Shaft v5 (Autodesk Fusion 360 design; units mm, degrees)
Autodesk Fusion 360 part; units mm, degrees
sketch "Sketch1" plane through (0, 0, 0) normal (0, 0, 1) x (1, 0, 0) in component "Normalny"
  circle A0 centre (0, 0) radius 6
  circle A1 centre (0, -1) radius 6 construction
  line L0 (0, 0) -> (0, -7) construction
  line L1 (0, 0) -> (-6, 0) construction
  line L2 (0, 0) -> (6, 0) construction
  circle A2 centre (-3, 0) radius 1.55
  circle A3 centre (3, 0) radius 1.55
  circle A4 centre (0, 0) radius 7
  dimension "d1" = 12
  dimension "d2" = 12
  dimension "d3" = 1
  dimension "d13" = 3.1
  dimension "d14" = 3.1
  dimension "d20" = 1
  dimension "d78" = 6
  dimension "d79" = 3
  constraint coincident A0.centre L0.start
  constraint coincident A0 L1.end
  constraint horizontal L1
  constraint coincident A0 L2.end
  constraint parallel L1 L2
  constraint coincident L1 A2.centre
  constraint coincident L2 A3.centre
  constraint perpendicular L0 L2
  measures "d1" diameter of A0
  measures "d2" diameter of A1
  measures "d3" distance of A0.centre A1.centre
  measures "d13" diameter of A2
  measures "d14" diameter of A3
  measures "d78" distance of A2.centre A3.centre
  measures "d79" distance of A0.centre A2.centre
extrude "Extrude1" add sketch "Sketch1" along normal blind 7 contours A0 makes body 1 in component "Normalny"
extrude "Extrude2" add sketch "Sketch1" along normal blind 3 contours A4 bodies 1 in component "Normalny"
sketch "Sketch1 (2)" plane through (0, 0, 0) normal (0, 0, -1) x (1, 0, 0) in component "Shifted"
  circle A0 centre (0, 0) radius 7
  circle A1 centre (-3, 0) radius 1.55
  circle A2 centre (3, 0) radius 1.55
  circle A3 centre (0, -1) radius 6
  line L0 (0, 0) -> (0, -3) construction
  dimension "d23" = 12
  dimension "d24" = 1
  constraint coincident A0.centre L0.start
  constraint vertical L0
  measures "d23" diameter of A3
  measures "d24" distance of A3.centre A0.centre
extrude "Extrude1'" add sketch "Sketch1 (2)" along normal blind 7 separate body contours A3 makes body 2 in component "Shifted"
sketch "Sketch2" plane through (0, 0, -7) normal (0, 0, -1) x (1, 0, 0) in component "Shifted"
  circle A0 centre (3, 0) radius 1.55
  circle A1 centre (-3, 0) radius 1.55
  circle A2 centre (0, -1) radius 6
  circle A3 centre (0, -1) radius 7
  dimension "d27" = 1
extrude "Extrude2'" add sketch "Sketch2" against normal blind 3 contours A3 bodies 2 in component "Shifted"
sketch "Sketch1 (3)" plane through (0, 0, -7) normal (0, 0, -1) x (1, 0, 0) in component "Shifted_2"
  circle A0 centre (0, -1) radius 7
  circle A1 centre (3, 0) radius 1.55
  circle A2 centre (-3, 0) radius 1.55
  line L0 (0, 0) -> (0, 4) construction
  circle A3 centre (0, 1) radius 6
  dimension "d30" = 12
  dimension "d31" = 1
  constraint coincident L0.start origin
  constraint vertical L0
  constraint coincident L0 A3.centre
  measures "d30" diameter of A3
  measures "d31" distance of L0.start A3.centre
extrude "Extrude1''" add sketch "Sketch1 (3)" along normal blind 7 separate body contours A0 A3 | A0 A3 picked at (0.1647, 2.697) picked at (0, 6.3217) makes body 3 in component "Shifted_2"
sketch "Sketch2 (2)" plane through (0, 0, -14) normal (0, 0, -1) x (1, 0, 0) in component "Shifted_2"
  circle A0 centre (-3, 0) radius 1.55
  circle A1 centre (3, 0) radius 1.55
  circle A2 centre (0, 1) radius 6
  circle A3 centre (0, 1) radius 7
  dimension "d73" = 1
extrude "Extrude2''" add sketch "Sketch2 (2)" against normal blind 3 contours A3 bodies 3 in component "Shifted_2"
sketch "Sketch1 (4)" plane through (0, 0, -14) normal (0, 0, -1) x (1, 0, 0) in component "normalny2"
  circle A0 centre (0, 0) radius 6
  circle A1 centre (0, 1) radius 7
  circle A2 centre (-3, 0) radius 1.55
  circle A3 centre (3, 0) radius 1.55
  dimension "d37" = 12
  constraint coincident A0.centre origin
  measures "d37" diameter of A0
extrude "Extrude1'''" add sketch "Sketch1 (4)" along normal blind 4 separate body contours A0 makes body 4 in component "normalny2"
sketch "Sketch2 (3)" plane through (0, 0, 0) normal (0, 0, -1) x (1, 0, 0) in component "Normalny"
  circle A0 centre (0, 0) radius 7
  circle A1 centre (-3, 0) radius 1.55
  circle A2 centre (3, 0) radius 1.55
  circle A3 centre (0, -1) radius 6
  circle A4 centre (0, -1) radius 7
  dimension "d40" = 1
sketch "Sketch3" plane through (0, 0, -7) normal (0, 0, -1) x (1, 0, 0) in component "Shifted"
  circle A0 centre (0, -1) radius 7
  circle A1 centre (3, 0) radius 1.55
  circle A2 centre (-3, 0) radius 1.55
  circle A3 centre (0, 1) radius 7
  circle A4 centre (0, 1) radius 6
  constraint concentric A3 A4
extrude "Extrude3" add sketch "Sketch3" along normal blind 3 contours A0 A3 A4 | A0 A3 A4 | A0 A4 | A0 A4 bodies 2 in component "Shifted"
extrude "Extrude3'" add sketch "Sketch2 (3)" along normal blind 3 contours A3 | A0 A4 | A0 A4 picked at (1.4828, 5.4862) picked at (0.6054, -7.293) bodies 1 in component "Normalny"
sketch "Sketch4" plane through (0, 0, -14) normal (0, 0, -1) x (1, 0, 0) in component "Shifted_2"
  circle A0 centre (0, 0) radius 6
  circle A1 centre (0, 0) radius 7
  circle A2 centre (0, 1) radius 7
  circle A3 centre (-3, 0) radius 1.55
  circle A4 centre (3, 0) radius 1.55
  dimension "d62" = 1
extrude "Extrude4" add sketch "Sketch4" along normal blind 3 contours A0 | A1 A2 | A1 A2 picked at (1.4828, 6.4862) picked at (0.6054, -6.293) bodies 3 in component "Shifted_2"
sketch "Sketch3 (2)" plane through (0, 0, 7) normal (0, 0, 1) x (-1, 0, 0) in component "Normalny"
  circle A0 centre (3, 0) radius 1.55
  circle A1 centre (-3, 0) radius 1.55
  circle A2 centre (0, 0) radius 6
  line L0 (-3, 0) -> (-3, 1.55) construction
  line L1 (-3.243, 1.5308) -> (-2.9975, 1.95)
  line L2 (-2.9975, 1.95) -> (-2.7592, 1.5312)
  line L3 (-3, 1.55) -> (-2.9975, 1.95) construction
  dimension "d80" = 30
  dimension "d81" = 30
  dimension "d82" = 0.4
  constraint coincident A1.centre L0.start
  constraint coincident A1 L0.end
  constraint vertical L0
  constraint coincident A1 L1.start
  constraint coincident A1 L2.end
  measures "d80" angle of L2 L3
  measures "d81" angle of L1 L3
  measures "d82" vertical distance of L0.end L1.end
extrude "Extrude4'" cut sketch "Sketch3 (2)" against normal blind 34 contours A1 L1 L2 bodies 1 in component "Normalny"
extrude "Extrude4''" cut sketch "Sketch3 (2)" against normal blind 34 contours A1 L1 L2 sketch seen with x (1, 0, 0) y (0, 1, 0) z (0, 0, 1) at (0, 0, 3) bodies 2 in component "Shifted"
extrude "Extrude5" cut sketch "Sketch3 (2)" against normal blind 34 contours A1 L1 L2 sketch seen with x (1, 0, 0) y (0, 1, 0) z (0, 0, 1) at (0, 0, 6) bodies 3 in component "Shifted_2"
extrude "Extrude2'''" cut sketch "Sketch3 (2)" against normal blind 34 contours A1 L1 L2 sketch seen with x (1, 0, 0) y (0, 1, 0) z (0, 0, 1) at (0, 0, 9) bodies 4 in component "normalny2"
component "Normalny" placed x (1, 0, 0) y (0, 1, 0) z (0, 0, 1) at (0, 0, 0)
component "Shifted" placed x (1, 0, 0) y (0, 1, 0) z (0, 0, 1) at (0, 0, -3)
component "Shifted_2" placed x (1, 0, 0) y (0, 1, 0) z (0, 0, 1) at (0, 0, -6)
component "normalny2" placed x (1, 0, 0) y (0, 1, 0) z (0, 0, 1) at (0, 0, -9)
equation "d79 = d78 / 2"
